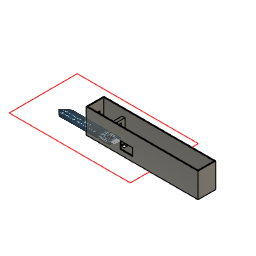
Case_moisture_sensor v2 (Autodesk Fusion 360 design; units mm, degrees)
Autodesk Fusion 360 part; units mm, degrees
sketch "Sketch1" plane through (0, 0, 0) normal (0, 0, 1) x (1, 0, 0)
  line L0 (95, -15) -> (-95, -15)
  line L1 (-95, -15) -> (-95, 15)
  line L2 (-95, 15) -> (95, 15)
  line L3 (95, 15) -> (95, -15)
  line L4 (95, -15) -> (-95, 15) construction
  line L5 (-95, -15) -> (95, 15) construction
  dimension "d3" = 190
  dimension "d4" = 30
  constraint horizontal L0
  constraint perpendicular L0 L1
  constraint parallel L0 L2
  constraint parallel L1 L3
  constraint coincident L4 origin
  constraint coincident L5 origin
  measures "d3" distance of L1.end L2.end
  measures "d4" distance of L0.end L1.end
extrude "Extrude1" add sketch "Sketch1" along normal blind 2
move_body "Move1" bodies 1 to x (1, 0, 0) y (0, 1, 0) z (0, 0, 1) at (90, -10, 0)
sketch "Sketch2" plane through (0, 0, 2) normal (0, 0, 1) x (-1, 0, 0)
  line L0 (-185, -5) -> (5, -5)
  line L1 (5, -5) -> (5, 25)
  line L2 (5, 25) -> (-185, 25)
  line L3 (-185, 25) -> (-185, -5)
  line L4 (-185, 10) -> (-175, 10)
  line L5 (-175, 0) -> (-175, 20)
  line L6 (-175, 20) -> (-99, 20)
  line L7 (-99, 20) -> (-99, 0)
  line L8 (-99, 0) -> (-175, 0)
  line L9 (-97, -2) -> (-177, -2)
  line L10 (-177, -2) -> (-177, 22)
  line L11 (-177, 22) -> (-97, 22)
  line L12 (-97, 22) -> (-97, -2)
  line L13 (-98, -1) -> (-176, -1)
  line L14 (-176, -1) -> (-176, 21)
  line L15 (-176, 21) -> (-98, 21)
  line L16 (-98, 21) -> (-98, -1)
  dimension "d7" = 10
  dimension "d8" = 76
  dimension "d9" = 5
  dimension "d10" = 5
  dimension "d11" = -2
  dimension "d12" = -1
  constraint midpoint L3 L4.start
  constraint perpendicular L3 L4
  constraint perpendicular L5 L6
  constraint parallel L5 L7
  constraint parallel L6 L8
  constraint perpendicular L2 L5
  measures "d7" distance of L4.start L4.end
  measures "d8" distance of L5.start L7.end
  measures "d9" distance of L0 L8
  measures "d10" distance of L2 L6
extrude "Extrude2" add sketch "Sketch2" along normal blind 10 contours L9 L10 L11 L12
sketch "Sketch3" plane through (0, 0, 2) normal (0, 0, 1) x (-1, 0, 0)
  line L0 (-185, -5) -> (5, -5)
  line L1 (5, -5) -> (5, 25)
  line L2 (5, 25) -> (-185, 25)
  line L3 (-185, 25) -> (-185, -5)
  line L4 (-97, 22) -> (-97, -2)
  line L5 (-97, -2) -> (-177, -2)
  line L6 (-177, -2) -> (-177, 22)
  line L7 (-177, 22) -> (-97, 22)
  line L8 (-183.5, -3.5) -> (3.5, -3.5)
  line L9 (3.5, -3.5) -> (3.5, 23.5)
  line L10 (3.5, 23.5) -> (-183.5, 23.5)
  line L11 (-183.5, 23.5) -> (-183.5, -3.5)
  dimension "d15" = -1.5
extrude "Extrude3" add sketch "Sketch3" along normal blind 40 contours L0 L1 L2 L3
sketch "Sketch4" plane through (-5, 0, 0) normal (-1, 0, 0) x (0, -1, 0)
  line L0 (-5, 0) -> (25, 0)
  line L1 (25, 0) -> (25, 42)
  line L2 (25, 42) -> (-5, 42)
  line L3 (-5, 42) -> (-5, 0)
  line L4 (22, 14.5) -> (-2, 14.5)
  line L5 (-2, 14.5) -> (-2, 17.5)
  line L6 (-2, 17.5) -> (22, 17.5)
  line L7 (22, 17.5) -> (22, 14.5)
  line L8 (22, 14.5) -> (-2, 17.5) construction
  line L9 (-2, 14.5) -> (22, 17.5) construction
  point P0 (10, 16)
  dimension "d18" = 24
  dimension "d19" = 3
  constraint horizontal L4
  constraint perpendicular L4 L5
  constraint parallel L4 L6
  constraint parallel L5 L7
  constraint coincident L8 P0
  constraint coincident L9 P0
  measures "d18" distance of L5.end L6.end
  measures "d19" distance of L4.end L5.end
extrude "Extrude4" cut sketch "Sketch4" against normal blind 4 contours L4 L5 L6 L7
sketch "Sketch5" plane through (-5, 0, 0) normal (-1, 0, 0) x (0, -1, 0)
  line L0 (-2, 14.5) -> (-2, 17.5)
  line L1 (-2, 17.5) -> (22, 17.5)
  line L2 (22, 17.5) -> (22, 14.5)
  line L3 (22, 14.5) -> (-2, 14.5)
  line L4 (-5, 0) -> (25, 0)
  line L5 (25, 0) -> (25, 42)
  line L6 (25, 42) -> (-5, 42)
  line L7 (-5, 42) -> (-5, 0)
  line L8 (10, 17.5) -> (10, 21.5)
  line L9 (17, 17.5) -> (3, 17.5)
  line L10 (3, 17.5) -> (3, 25.5)
  line L11 (3, 25.5) -> (17, 25.5)
  line L12 (17, 25.5) -> (17, 17.5)
  line L13 (17, 17.5) -> (3, 25.5) construction
  line L14 (3, 17.5) -> (17, 25.5) construction
  point P0 (10, 21.5)
  dimension "d22" = 4
  dimension "d23" = 14
  dimension "d24" = 8
  constraint midpoint L1 L8.start
  constraint perpendicular L1 L8
  constraint horizontal L9
  constraint perpendicular L9 L10
  constraint parallel L9 L11
  constraint parallel L10 L12
  constraint coincident L13 P0
  constraint coincident L14 P0
  constraint coincident P0 L8.end
  measures "d22" distance of L8.start P0
  measures "d23" distance of L10.end L11.end
  measures "d24" distance of L9.end L10.end
extrude "Extrude5" cut sketch "Sketch5" against normal blind 57 contours L1 L9 L10 L11 L12
sketch "Sketch6" plane through (0, 0, 2) normal (0, 0, 1) x (-1, 0, 0)
  line L0 (-183.5, -3.5) -> (3.5, -3.5)
  line L1 (3.5, -3.5) -> (3.5, 23.5)
  line L2 (3.5, 23.5) -> (-183.5, 23.5)
  line L3 (-183.5, 23.5) -> (-183.5, -3.5)
  line L4 (-97, 22) -> (-97, -2)
  line L5 (-97, -2) -> (-177, -2)
  line L6 (-177, -2) -> (-177, 22)
  line L7 (-177, 22) -> (-97, 22)
  line L8 (-27.625, 23.5) -> (-32.625, 23.5)
  line L9 (-32.625, 23.5) -> (-32.625, -3.5)
  line L10 (-32.625, -3.5) -> (-27.625, -3.5)
  line L11 (-27.625, -3.5) -> (-27.625, 23.5)
  dimension "d27" = 5
  constraint horizontal L8
  constraint vertical L9
  constraint horizontal L10
  constraint vertical L11
  constraint coincident L2 L8.start
  measures "d27" distance of L8.start L8.end
extrude "Extrude6" add sketch "Sketch6" along normal blind 28 contours L0 L2 L8 L9 L10 L11
extrude "Extrude7" cut sketch "Sketch5" against normal blind 41 contours L1 L9 L10 L11 L12
sketch "Sketch7" plane through (-3.5, 0, 0) normal (1, 0, 0) x (0, 1, 0)
  line L0 (-23.5, 2) -> (3.5, 2)
  line L1 (3.5, 2) -> (3.5, 42)
  line L2 (3.5, 42) -> (-23.5, 42)
  line L3 (-23.5, 42) -> (-23.5, 2)
  line L4 (-17, 17.5) -> (-17, 25.5)
  line L5 (-17, 25.5) -> (-3, 25.5)
  line L6 (-3, 25.5) -> (-3, 17.5)
  line L7 (-3, 17.5) -> (2, 17.5)
  line L8 (2, 17.5) -> (2, 14.5)
  line L9 (2, 14.5) -> (-22, 14.5)
  line L10 (-22, 14.5) -> (-22, 17.5)
  line L11 (-22, 17.5) -> (-17, 17.5)
  line L12 (-22, 14.5) -> (2, 14.5)
  line L13 (2, 14.5) -> (2, 11.5)
  line L14 (2, 11.5) -> (-22, 11.5)
  line L15 (-22, 11.5) -> (-22, 14.5)
  dimension "d32" = 3
  constraint horizontal L12
  constraint vertical L13
  constraint horizontal L14
  constraint vertical L15
  constraint coincident L9.end L10.start
  measures "d32" distance of L9.end L14.end
extrude "Extrude8" add sketch "Sketch7" along normal blind 31.125 contours L9 L12 L13 L14 L15
sketch "Sketch8" plane through (0, -25, 0) normal (0, -1, 0) x (1, 0, 0)
  line L0 (-5, 0) -> (185, 0)
  line L1 (185, 0) -> (185, 42)
  line L2 (185, 42) -> (-5, 42)
  line L3 (-5, 42) -> (-5, 0)
  line L4 (53, 0) -> (53, 42)
  line L5 (53, 21) -> (74, 21)
  line L6 (74, 21) -> (74, 8)
  line L7 (74, 8) -> (53, 8)
  line L8 (53, 8) -> (53, 21)
  dimension "d35" = 21
  dimension "d36" = 13
  constraint coincident L0 L4.start
  constraint coincident L2 L4.end
  constraint perpendicular L2 L4
  constraint horizontal L5
  constraint vertical L6
  constraint horizontal L7
  constraint vertical L8
  constraint midpoint L4 L5.start
  measures "d35" distance of L5.start L5.end
  measures "d36" distance of L5.start L7.end
extrude "Extrude9" cut sketch "Sketch8" against normal blind 2 contours L4 L5 L6 L7 L8
sketch "Sketch9" plane through (0, 5, 0) normal (0, 1, 0) x (-1, 0, 0)
  line L0 (-185, 0) -> (5, 0)
  line L1 (5, 0) -> (5, 42)
  line L2 (5, 42) -> (-185, 42)
  line L3 (-185, 42) -> (-185, 0)
  line L4 (-77, 4) -> (-94, 4)
  line L5 (-94, 4) -> (-94, 14)
  line L6 (-94, 14) -> (-77, 14)
  line L7 (-77, 14) -> (-77, 4)
  dimension "d39" = 17
  dimension "d40" = 10
  constraint horizontal L4
  constraint vertical L5
  constraint horizontal L6
  constraint vertical L7
  measures "d39" distance of L4.start L4.end
  measures "d40" distance of L4.start L6.end
extrude "Extrude10" cut sketch "Sketch9" against normal blind 2 contours L4 L5 L6 L7
sketch "Sketch10" plane through (0, 0, 0) normal (0, 0, -1) x (1, 0, 0)
  line L0 (-5, -5) -> (185, -5)
  line L1 (185, -5) -> (185, 25)
  line L2 (185, 25) -> (-5, 25)
  line L3 (-5, 25) -> (-5, -5)
  line L4 (34, 18.5) -> (46, 18.5)
  line L5 (46, 18.5) -> (46, 1.5)
  line L6 (46, 1.5) -> (34, 1.5)
  line L7 (34, 1.5) -> (34, 18.5)
  line L8 (46, 10) -> (44.75, 10)
  line L9 (48, 6.75) -> (41.5, 6.75)
  line L10 (41.5, 6.75) -> (41.5, 13.25)
  line L11 (41.5, 13.25) -> (48, 13.25)
  line L12 (48, 13.25) -> (48, 6.75)
  line L13 (48, 6.75) -> (41.5, 13.25) construction
  line L14 (41.5, 6.75) -> (48, 13.25) construction
  point P0 (44.75, 10)
  dimension "d43" = 12
  dimension "d44" = 17
  dimension "d45" = 6.5
  dimension "d46" = 5
  dimension "d47" = 6.5
  dimension "d48" = 6.5
  constraint horizontal L4
  constraint vertical L5
  constraint horizontal L6
  constraint vertical L7
  constraint midpoint L5 L8.start
  constraint perpendicular L5 L8
  constraint horizontal L9
  constraint perpendicular L9 L10
  constraint parallel L9 L11
  constraint parallel L10 L12
  constraint coincident L13 P0
  constraint coincident L14 P0
  constraint coincident P0 L8.end
  measures "d43" distance of L4.start L4.end
  measures "d44" distance of L4.start L6.end
  measures "d45" distance of L2 L4
  measures "d47" distance of L10.end L11.end
  measures "d48" distance of L9.end L10.end
extrude "Extrude11" cut sketch "Sketch10" against normal blind 2 contours L5 L9 L11 L12 | L5 L9 L10 L11
sketch "Sketch11" plane through (176, 0, 0) normal (-1, 0, 0) x (0, -1, 0)
  line L0 (-1, 2) -> (21, 2)
  line L1 (21, 2) -> (21, 12)
  line L2 (21, 12) -> (-1, 12)
  line L3 (-1, 12) -> (-1, 2)
  line L4 (-1, 2) -> (3, 2)
  line L5 (3, 2) -> (3, 12)
  line L6 (3, 12) -> (-1, 12)
  line L7 (-1, 12) -> (-1, 2)
  dimension "d51" = 4
  constraint horizontal L4
  constraint vertical L5
  constraint horizontal L6
  constraint vertical L7
  constraint coincident L0.start L3.end
  measures "d51" distance of L0.start L4.end
extrude "Extrude12" cut sketch "Sketch11" against normal blind 1 contours L0 L2 L3 L4 L5 L6 L7
sketch "Sketch12" plane through (98, 0, 0) normal (1, 0, 0) x (0, 1, 0)
  line L0 (-21, 2) -> (1, 2)
  line L1 (1, 2) -> (1, 12)
  line L2 (1, 12) -> (-21, 12)
  line L3 (-21, 12) -> (-21, 2)
  line L4 (-21, 2) -> (-17, 2)
  line L5 (-17, 2) -> (-17, 12)
  line L6 (-17, 12) -> (-21, 12)
  line L7 (-21, 12) -> (-21, 2)
  dimension "d54" = 4
  constraint horizontal L4
  constraint vertical L5
  constraint horizontal L6
  constraint vertical L7
  constraint coincident L0.start L3.end
  measures "d54" distance of L0.start L4.end
extrude "Extrude13" cut sketch "Sketch12" against normal blind 1 contours L0 L2 L3 L4 L5 L6 L7
equation "d16 = 30 mm + 10 mm"
equation "d28 = 30.00 mm - 2 mm"
equation "d35 = 19 mm + 2 mm"
equation "d36 = 12 mm + 1 mm"
equation "d39 = 15 mm + 2 mm"
equation "d45 = 8 mm - 1.5 mm"
